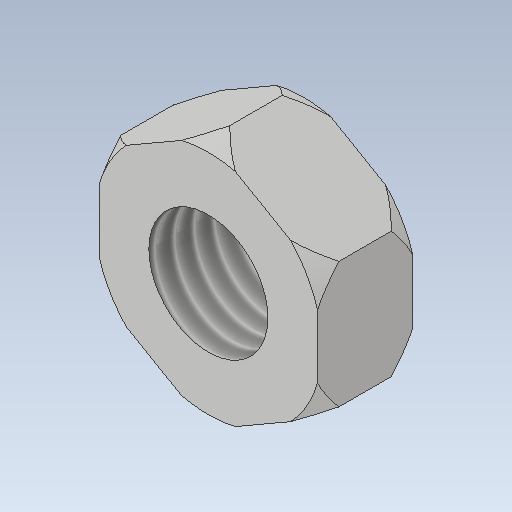
# Autodesk Inventor part: Гайка М3
Saved by Autodesk Inventor 2020 (Build 240168000, 168)
## iProperties
Created: 2020-03-17
Part Number: Гайка М3
Material: Типовые
Document SubType Name: Modeling
Designer: Leancher
Density: 1 g/cm^3
Appearance: По умолчанию
Author: Leancher
Autodesk Inventor part; units mm, degrees
ref_plane "YZ Plane" through (0, 0, 0) normal (1, 0, 0) x (0, 1, 0)
ref_plane "XZ Plane" through (0, 0, 0) normal (0, 1, 0) x (-1, 0, 0)
ref_plane "XY Plane" through (0, 0, 0) normal (0, 0, 1) x (1, 0, 0)
sketch "Эскиз1" plane through (0, 0, 0) normal (0, 1, 0) x (-1, 0, 0)
  line L0 (0, 0) -> (0, 2.4)
  line L1 (0, 2.4) -> (-2.8635, 2.4)
  line L2 (-2.8635, 0) -> (0, 0)
  line L3 (0, 1.2) -> (-4.2844, 1.2) construction
  line L4 (-2.8635, 0) -> (-3.176, 0.5413)
  line L5 (-2.8635, 2.4) -> (-3.176, 1.8587)
  line L6 (-3.176, 1.8587) -> (-3.176, 0.5413)
  constraints: 14 end point, 1 horizontal, 1 midpoint
revolve "Вращение1" add sketch "Эскиз1" angle 360 about axis through (0, 0, 0) along (0, 0, 1)
sketch "Эскиз2" plane through (0, 0, 2.4) normal (0, 0, 1) x (1, 0, 0)
  circle A0 centre (0, 0) radius 1.5
  line L0 (2.75, -1.5877) -> (2.75, 1.5877)
  line L1 (-2.75, -1.5877) -> (-2.75, 1.5877)
  line L2 (0, 3.1754) -> (2.75, 1.5877)
  line L3 (0, 3.1754) -> (-2.75, 1.5877)
  line L4 (-2.75, -1.5877) -> (0, -3.1754)
  line L5 (0, -3.1754) -> (2.75, -1.5877)
  constraints: 12 end point, 1 centre point
extrude "Выдавливание1" cut sketch "Эскиз2" against normal blind 2.4 keep common part
thread "Резьба1" size "M3x0.5" class "6H" standard "ANSI Metric M Profile" full length
